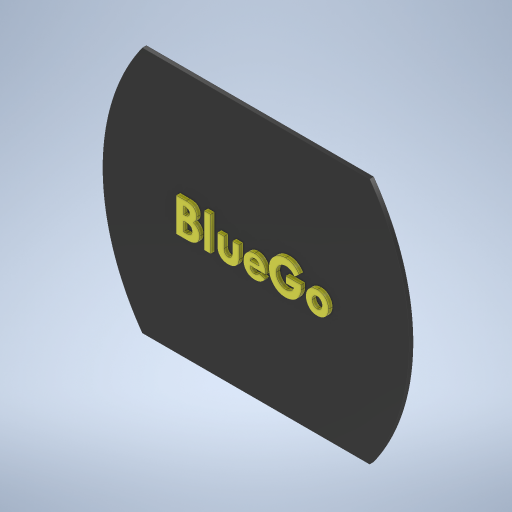
# Autodesk Inventor part: BlueGo
Saved by Autodesk Inventor 2024.3 (Build 283343000, 343)
## iProperties
Created: 2025-11-11
Part Number: BlueGo
Material: Generic
Document SubType Name: Modeling
Designer: tizia
Density: 1 g/cm^3
Appearance: White
Author: tizia
Autodesk Inventor part; units mm, degrees
ref_plane "YZ Plane" through (0, 0, 0) normal (1, 0, 0) x (0, 1, 0)
ref_plane "XZ Plane" through (0, 0, 0) normal (0, 1, 0) x (-1, 0, 0)
ref_plane "XY Plane" through (0, 0, 0) normal (0, 0, 1) x (1, 0, 0)
sketch "Sketch1" plane through (0, 0, 0) normal (0, 0, 1) x (1, 0, 0)
  line L0 (57.5, 62.5) -> (-57.5, 62.5)
  line L1 (-57.5, 62.5) -> (-57.5, -62.5)
  line L2 (-57.5, -62.5) -> (57.5, -62.5)
  line L3 (57.5, -62.5) -> (57.5, 62.5)
  line L4 (57.5, 62.5) -> (-57.5, -62.5) construction
  line L5 (-57.5, 62.5) -> (57.5, -62.5) construction
  line L6 (57.5, 0) -> (77.5, 0)
  line L7 (-57.5, 0) -> (-77.5, 0)
  arc A0 (-57.5, 62.5) -> (-57.5, -62.5) centre (30.1562, 0) ccw
  arc A1 (57.5, -62.5) -> (57.5, 62.5) centre (-30.1562, 0) ccw
  point P0 (0, 0)
  dimension "d0" = 115
  dimension "d1" = 125
  dimension "d2" = 20
  dimension "d3" = 20
  constraints: 16 end point, 6 point on circle, 4 midpoint, 3 horizontal, 2 centre point, 2 parallel, 1 perpendicular
  measures "d0" distance of L2.end L1.end
  measures "d1" distance of L1.end L0.end
  measures "d2" distance of L6.start L6.end
  measures "d3" distance of L7.start L7.end
extrude "Extrusion1" add sketch "Sketch1" along normal blind 2
sketch "Sketch2" plane through (0, 0, 2) normal (0, 0, 1) x (1, 0, 0)
  line L0 (-40.012, 8.7608) -> (40.012, 8.7608) construction
  line L1 (40.012, 8.7608) -> (40.012, -8.7608) construction
  line L2 (40.012, -8.7608) -> (-40.012, -8.7608) construction
  line L3 (-40.012, -8.7608) -> (-40.012, 8.7608) construction
  line L4 (-38.3346, 8.4789) -> (-33.3727, 8.4789)
  spline S0 degree 2 poles (-33.3727, 8.4789) (-30.2716, 8.4789) (-27.988, 5.8852) (-27.988, 4.1513) knots 0 0 0 1 2 2 2
  spline S1 degree 2 poles (-27.988, 4.1513) (-27.988, 3.0518) (-28.8197, 1.5435) (-29.7359, 0.7682) knots 0 0 0 1 2 2 2
  spline S2 degree 2 poles (-29.7359, 0.7682) (-27.9739, 0.148) (-26.5079, -2.2201) (-26.5079, -3.5593) knots 0 0 0 1 2 2 2
  spline S3 degree 2 poles (-26.5079, -3.5593) (-26.5079, -5.8993) (-29.7218, -8.5211) (-32.6397, -8.5211) knots 0 0 0 1 2 2 2
  line L5 (-32.6397, -8.5211) -> (-38.3346, -8.5211)
  line L6 (-38.3346, -8.5211) -> (-38.3346, 8.4789)
  line L7 (-34.6696, -0.9938) -> (-34.6696, -5.6737)
  line L8 (-34.6696, -5.6737) -> (-33.3445, -5.6737)
  spline S4 degree 2 poles (-33.3445, -5.6737) (-30.3279, -5.6737) (-30.3279, -3.4747) knots 0 0 0 1 1 1
  spline S5 degree 2 poles (-30.3279, -3.4747) (-30.3279, -2.2765) (-31.7939, -0.9938) (-33.1754, -0.9938) knots 0 0 0 1 2 2 2
  line L9 (-33.1754, -0.9938) -> (-34.6696, -0.9938)
  line L10 (-34.6696, 5.6314) -> (-34.6696, 1.8959)
  line L11 (-34.6696, 1.8959) -> (-33.8238, 1.8959)
  spline S6 degree 2 poles (-33.8238, 1.8959) (-32.8935, 1.8959) (-31.6248, 3.08) (-31.6248, 3.954) knots 0 0 0 1 2 2 2
  spline S7 degree 2 poles (-31.6248, 3.954) (-31.6248, 4.6588) (-32.8653, 5.6314) (-33.7956, 5.6314) knots 0 0 0 1 2 2 2
  line L12 (-33.7956, 5.6314) -> (-34.6696, 5.6314)
  line L13 (-24.2384, 8.7608) -> (-20.9258, 8.7608)
  line L14 (-20.9258, 8.7608) -> (-20.9258, -8.5211)
  line L15 (-20.9258, -8.5211) -> (-24.2384, -8.5211)
  line L16 (-24.2384, -8.5211) -> (-24.2384, 8.7608)
  line L17 (-17.5145, 2.5867) -> (-14.1455, 2.5867)
  line L18 (-14.1455, 2.5867) -> (-14.1455, -2.7558)
  spline S8 degree 2 poles (-14.1455, -2.7558) (-14.1455, -3.9117) (-12.9755, -5.4482) (-12.1157, -5.4482) knots 0 0 0 1 2 2 2
  spline S9 degree 2 poles (-12.1157, -5.4482) (-11.1994, -5.4482) (-9.9449, -3.954) (-9.9449, -2.8263) knots 0 0 0 1 2 2 2
  line L19 (-9.9449, -2.8263) -> (-9.9449, 2.5867)
  line L20 (-9.9449, 2.5867) -> (-6.5759, 2.5867)
  line L21 (-6.5759, 2.5867) -> (-6.5759, -3.8835)
  spline S10 degree 2 poles (-6.5759, -3.8835) (-6.5759, -5.9415) (-9.7193, -8.7326) (-12.0593, -8.7326) knots 0 0 0 1 2 2 2
  spline S11 degree 2 poles (-12.0593, -8.7326) (-14.5402, -8.7326) (-17.5145, -5.9415) (-17.5145, -3.6157) knots 0 0 0 1 2 2 2
  line L22 (-17.5145, -3.6157) -> (-17.5145, 2.5867)
  line L23 (6.9424, -3.7566) -> (-0.9938, -3.7566)
  spline S12 degree 2 poles (-0.9938, -3.7566) (-0.9233, -4.8279) (0.3595, -6.1671) (1.2052, -6.1671) knots 0 0 0 1 2 2 2
  spline S13 degree 2 poles (1.2052, -6.1671) (2.7417, -6.1671) (3.6016, -4.7857) knots 0 0 0 1 1 1
  line L24 (3.6016, -4.7857) -> (6.6464, -5.8006)
  spline S14 degree 2 poles (6.6464, -5.8006) (4.9548, -8.7608) (1.3744, -8.7608) knots 0 0 0 1 1 1
  spline S15 degree 2 poles (1.3744, -8.7608) (-1.2475, -8.7608) (-4.3628, -5.575) (-4.3628, -2.8827) knots 0 0 0 1 2 2 2
  spline S16 degree 2 poles (-4.3628, -2.8827) (-4.3628, -0.4581) (-1.0925, 2.8263) (1.3039, 2.8263) knots 0 0 0 1 2 2 2
  spline S17 degree 2 poles (1.3039, 2.8263) (3.7143, 2.8263) (6.9424, -0.6273) (6.9424, -3.221) knots 0 0 0 1 2 2 2
  line L25 (6.9424, -3.221) -> (6.9424, -3.7566)
  line L26 (-0.9656, -1.5294) -> (3.517, -1.5294)
  spline S18 degree 2 poles (3.517, -1.5294) (3.0518, 0.5568) (1.3744, 0.5568) knots 0 0 0 1 1 1
  spline S19 degree 2 poles (1.3744, 0.5568) (0.4158, 0.5568) (-0.8387, -0.5286) (-0.9656, -1.5294) knots 0 0 0 1 2 2 2
  line L27 (23.8719, 4.7857) -> (21.4332, 2.5021)
  spline S20 degree 2 poles (21.4332, 2.5021) (20.6721, 3.813) (18.4167, 5.124) (17.1903, 5.124) knots 0 0 0 1 2 2 2
  spline S21 degree 2 poles (17.1903, 5.124) (15.2027, 5.124) (12.2566, 2.0933) (12.2566, 0.0493) knots 0 0 0 1 2 2 2
  spline S22 degree 2 poles (12.2566, 0.0493) (12.2566, -2.1356) (15.1886, -5.1803) (17.2608, -5.1803) knots 0 0 0 1 2 2 2
  spline S23 degree 2 poles (17.2608, -5.1803) (18.3885, -5.1803) (20.4747, -4.0386) (21.109, -2.4739) knots 0 0 0 1 2 2 2
  line L28 (21.109, -2.4739) -> (17.0775, -2.4739)
  line L29 (17.0775, -2.4739) -> (17.0775, 0.8387)
  line L30 (17.0775, 0.8387) -> (24.9291, 0.8387)
  line L31 (24.9291, 0.8387) -> (24.9291, -1.3603)
  spline S24 degree 2 poles (24.9291, -1.3603) (24.9291, -3.0659) (22.6032, -6.9565) (18.7973, -8.7608) (16.852, -8.7608) knots 0 0 0 1 2 3 3 3
  spline S25 degree 2 poles (16.852, -8.7608) (13.3279, -8.7608) (8.493, -3.658) (8.493, 0.0916) knots 0 0 0 1 2 2 2
  spline S26 degree 2 poles (8.493, 0.0916) (8.493, 3.658) (13.483, 8.7044) (16.9789, 8.7044) knots 0 0 0 1 2 2 2
  spline S27 degree 2 poles (16.9789, 8.7044) (21.4614, 8.7044) (23.8719, 4.7857) knots 0 0 0 1 1 1
  spline S28 degree 2 poles (27.2127, -2.9813) (27.2127, -0.4017) (30.4971, 2.8545) (33.0767, 2.8545) knots 0 0 0 1 2 2 2
  spline S29 degree 2 poles (33.0767, 2.8545) (35.4731, 2.8545) (38.7152, -0.4722) (38.7152, -2.9391) knots 0 0 0 1 2 2 2
  spline S30 degree 2 poles (38.7152, -2.9391) (38.7152, -5.4482) (35.4731, -8.7608) (33.0203, -8.7608) knots 0 0 0 1 2 2 2
  spline S31 degree 2 poles (33.0203, -8.7608) (30.2716, -8.7608) (27.2127, -5.2508) (27.2127, -2.9813) knots 0 0 0 1 2 2 2
  spline S32 degree 2 poles (35.459, -2.9813) (35.459, -1.8536) (33.9789, -0.1762) (32.9921, -0.1762) knots 0 0 0 1 2 2 2
  spline S33 degree 2 poles (32.9921, -0.1762) (31.9772, -0.1762) (30.4971, -1.755) (30.4971, -2.8545) knots 0 0 0 1 2 2 2
  spline S34 degree 2 poles (30.4971, -2.8545) (30.4971, -4.0667) (31.9631, -5.7442) (32.9921, -5.7442) knots 0 0 0 1 2 2 2
  spline S35 degree 2 poles (32.9921, -5.7442) (33.9789, -5.7442) (35.459, -4.0949) (35.459, -2.9813) knots 0 0 0 1 2 2 2
  point P0 (0, 0)
  constraints: 2 other
extrude "Extrusion2" add sketch "Sketch2" along normal blind 2
sketch "Sketch3" plane through (-38.3346, -8.5211, 2) normal (-1, 0, 0) x (0, 0, 1)
  point P0 (-2, 8.5211)
body "Solid1"
